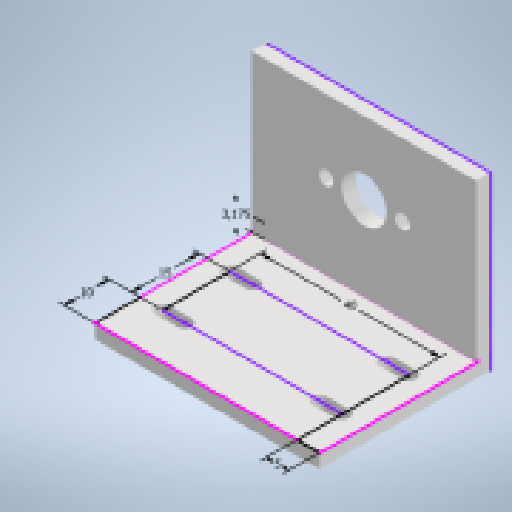
# Autodesk Inventor part: Suportepara o motor em cantorneira
Saved by Autodesk Inventor 2023 (Build 270158000, 158)
## iProperties
Created: 2022-10-11
Part Number: Suportepara o motor em cantorneira
Material: Generic
Document SubType Name: Modeling
Designer: klebe
Density: 1 g/cm^3
Appearance: Default
Description: Suporte em aço astm A36 - 1.1/2 x 1/8
Author: klebe
Autodesk Inventor part; units mm, degrees
ref_plane "YZ Plane" through (0, 0, 0) normal (1, 0, 0) x (0, 1, 0)
ref_plane "XZ Plane" through (0, 0, 0) normal (0, 1, 0) x (-1, 0, 0)
ref_plane "XY Plane" through (0, 0, 0) normal (0, 0, 1) x (1, 0, 0)
sketch "Sketch1" plane through (0, 0, 0) normal (0, 0, 1) x (1, 0, 0)
  line L0 (25, 16.8) -> (25, -19.8)
  line L1 (25, -19.8) -> (-25, -19.8)
  line L2 (-25, -19.8) -> (-25, 16.8)
  line L3 (-25, -19.8) -> (-25, -16.8)
  line L4 (-25, -19.8) -> (-25, 18.3)
  line L5 (-25, 18.3) -> (25, 18.3)
  line L6 (25, 18.3) -> (25, -19.8)
  line L7 (-25, -19.8) -> (-25, -16.625)
  line L8 (-25, -16.625) -> (25, -16.625)
  dimension "d94" = 3.175
  constraints: 18 end point, 3 point on line, 1 collinear, 1 horizontal, 1 parallel, 1 perpendicular, 1 vertical
  measures "d94" distance of L1.end L7.end
extrude "Extrusion3" add sketch "Sketch1" along normal blind 3.175
extrude "Extrusion4" add sketch "Sketch1" along normal blind 38.1 contours L0 L1 L2 L8
sketch "Sketch2" plane through (-25, -16.625, 3) normal (0, 1, 0) x (1, 0, 0)
  line L0 (50, -35.1) -> (0, -35.1) projected
  line L1 (0, 0) -> (50, 0) projected
  line L2 (0, 0) -> (0, -35.1) projected
  line L3 (50, 0) -> (50, -35.1) projected
  line L4 (50, -35.1) -> (45, -35.1)
  line L5 (0, -35.1) -> (0, -25.1)
  line L6 (0, 3) -> (0, -35.1) projected
  line L7 (45, -35.1) -> (45, -25.1)
  line L8 (45, -25.1) -> (5, -25.1)
  line L9 (5, -25.1) -> (5, -10.1)
  line L10 (5, -10.1) -> (45, -10.1)
  line L11 (45, -10.1) -> (45, -25.1)
  point P0 (40, -25.1)
  point P1 (40, -10)
  point P2 (10, -10)
  point P3 (10, -25.1)
  dimension "d83" = 5
  dimension "d84" = 10
  dimension "d85" = 40
  dimension "d86" = 15
  constraints: 14 end point, 2 parallel, 2 point on line, 1 horizontal, 1 perpendicular, 1 vertical
  measures "d83" distance of L0.start L4.end
  measures "d84" distance of L0.end L5.end
  measures "d85" distance of L9.end L10.end
  measures "d86" distance of L8.end L9.end
sketch "Sketch3" plane through (0, 0, 0) normal (0, 0, -1) x (-1, 0, 0)
  line L0 (25, 18.3) -> (25, -0.75)
  line L1 (-25, -16.8) -> (-25, 18.3) projected
  line L2 (25, 18.3) -> (25, 2.3)
  line L3 (25, 18.3) -> (25, -19.8) projected
  line L4 (0, 2.2) -> (0.1, 2.2)
  point P0 (0, -0.75)
  dimension "d67" = 19.05
  dimension "d68" = 25
  dimension "d95" = 16
  dimension "d98" = 0.1
  constraints: 6 end point, 1 point on line, 1 vertical
  measures "d67" distance of L0.start L0.end
  measures "d68" distance of L0.end point (0, -0.75)
  measures "d95" distance of L0.start L2.end
  measures "d98" distance of L4.start L4.end
hole "Hole4" at (0, 2.2, 0) direction (0, 0, 1) diameter 10 end through all
sketch "Sketch4" plane through (0, 0, 0) normal (0, 0, -1) x (-1, 0, 0)
  circle A0 centre (-8.5, 2.2) radius 1.2295 projected
  circle A1 centre (8.5, 2.2) radius 1.2295 projected
  line L0 (-25, 18.3) -> (25, 18.3) projected
  line L1 (25, 18.3) -> (25, 2.3)
  line L2 (25, 18.3) -> (25, -19.8) projected
  line L3 (8.5, 2.2) -> (-8.5, 2.1769)
  point P0 (0, 0)
  point P1 (8.5, 2.1769)
  dimension "d96" = 16
  constraints: 4 end point, 1 point on line
  measures "d96" distance of L0.end L1.end
hole "Hole5" at (8.5, 2.1769, 0) at (-8.5, 2.1769, 0) direction (0, 0, 1) diameter 3.18 end through all
sketch "Sketch5" plane through (-25, -16.625, 3.175) normal (0, 1, 0) x (1, 0, 0)
  arc A0 (45, -26.515) -> (45, -23.335) centre (45, -24.925) ccw
  arc A1 (40, -23.335) -> (40, -26.515) centre (40, -24.925) ccw
  line L0 (45, -26.515) -> (40, -26.515)
  line L1 (40, -23.335) -> (45, -23.335)
  arc A2 (45, -11.515) -> (45, -8.335) centre (45, -9.925) ccw
  arc A3 (40, -8.335) -> (40, -11.515) centre (40, -9.925) ccw
  line L2 (45, -11.515) -> (40, -11.515)
  line L3 (40, -8.335) -> (45, -8.335)
  arc A4 (10, -26.515) -> (10, -23.335) centre (10, -24.925) ccw
  arc A5 (5, -23.335) -> (5, -26.515) centre (5, -24.925) ccw
  line L4 (10, -26.515) -> (5, -26.515)
  line L5 (5, -23.335) -> (10, -23.335)
  arc A6 (10, -11.515) -> (10, -8.335) centre (10, -9.925) ccw
  arc A7 (5, -8.335) -> (5, -11.515) centre (5, -9.925) ccw
  line L6 (10, -11.515) -> (5, -11.515)
  line L7 (5, -8.335) -> (10, -8.335)
  point P0 (25, 3.175)
  constraints: 16 end point, 16 point on circle, 8 centre point, 7 tangent
extrude "Extrusion5" cut sketch "Sketch5" against normal blind 10
body "Solid2"
